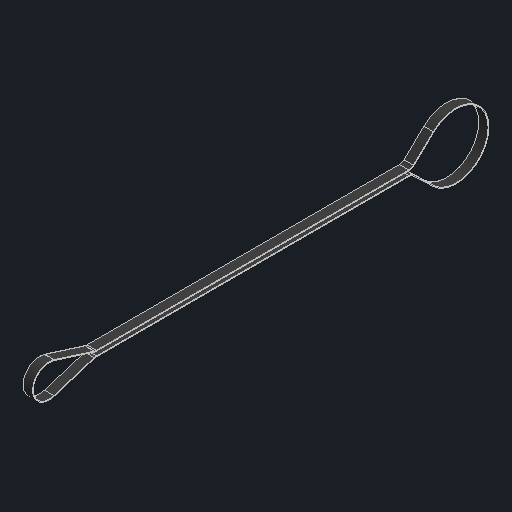
# Autodesk Inventor part: scara-belt3
Saved by Autodesk Inventor 2022 (Build 260153000, 153)
## iProperties
Created: 2021-07-18
Part Number: scara-belt3
Material: ゴム
Document SubType Name: Modeling
Designer: yuta0
Density: 0.93 g/cm^3
Appearance: ゴム - 黒
Mass: 8.55769 g
Surface Area: 248.449 cm^2
Volume: 9.20182 cm^3
Description: 在庫有
購入先: ミスミ
在庫数: 0.0
Author: yuta0
Autodesk Inventor part; units mm, degrees
ref_plane "YZ Plane" through (0, 0, 0) normal (1, 0, 0) x (0, 1, 0)
ref_plane "XZ Plane" through (0, 0, 0) normal (0, 1, 0) x (-1, 0, 0)
ref_plane "XY Plane" through (0, 0, 0) normal (0, 0, 1) x (1, 0, 0)
sketch "スケッチ1" plane through (0, 0, 0) normal (1, 0, 0) x (0, 1, 0)
  arc A0 (16.3891, -5.1817) -> (-16.3891, -5.1817) centre (0, 0) ccw
  arc A1 (-24.8353, -406.9299) -> (24.8353, -406.9299) centre (0, -430.7) ccw
  arc A2 (-2.581, -50) -> (-2.9261, -47.7635) centre (-10, -50) ccw
  line L0 (-2.9261, -47.7635) -> (-16.3891, -5.1817)
  line L1 (16.3891, -5.1817) -> (2.9261, -47.7635)
  line L2 (24.8353, -406.9299) -> (4.6403, -385.8298)
  line L3 (-24.8353, -406.9299) -> (-4.6403, -385.8298)
  arc A3 (2.9261, -47.7635) -> (2.581, -50) centre (10, -50) ccw
  arc A4 (2.581, -380.7) -> (4.6403, -385.8298) centre (10, -380.7) ccw
  arc A5 (-4.6403, -385.8298) -> (-2.581, -380.7) centre (-10, -380.7) ccw
  line L4 (-2.581, -50) -> (-2.581, -380.7)
  line L5 (2.581, -380.7) -> (2.581, -50)
  line L6 (3.3256, -47.8898) -> (16.7886, -5.308)
  arc A6 (16.7886, -5.308) -> (-16.7886, -5.308) centre (0, 0) ccw
  line L7 (-16.7886, -5.308) -> (-3.3256, -47.8898)
  arc A7 (-3, -50) -> (-3.3256, -47.8898) centre (-10, -50) ccw
  line L8 (-3, -50) -> (-3, -380.7)
  arc A8 (-4.943, -385.5401) -> (-3, -380.7) centre (-10, -380.7) ccw
  line L9 (-4.943, -385.5401) -> (-25.138, -406.6402)
  arc A9 (-25.138, -406.6402) -> (25.138, -406.6402) centre (0, -430.7) ccw
  line L10 (25.138, -406.6402) -> (4.943, -385.5401)
  arc A10 (3, -380.7) -> (4.943, -385.5401) centre (10, -380.7) ccw
  line L11 (3, -380.7) -> (3, -50)
  arc A11 (3.3256, -47.8898) -> (3, -50) centre (10, -50) ccw
  arc A12 (2.5629, -47.6486) -> (2.2, -50) centre (10, -50) ccw
  line L12 (2.5629, -47.6486) -> (16.0258, -5.0668)
  arc A13 (16.0258, -5.0668) -> (-16.0258, -5.0668) centre (0, 0) ccw
  line L13 (-16.0258, -5.0668) -> (-2.5629, -47.6486)
  arc A14 (-2.2, -50) -> (-2.5629, -47.6486) centre (-10, -50) ccw
  line L14 (-2.2, -50) -> (-2.2, -380.7)
  arc A15 (-4.365, -386.0933) -> (-2.2, -380.7) centre (-10, -380.7) ccw
  line L15 (-4.365, -386.0933) -> (-24.5601, -407.1934)
  arc A16 (-24.5601, -407.1934) -> (24.5601, -407.1934) centre (0, -430.7) ccw
  line L16 (24.5601, -407.1934) -> (4.365, -386.0933)
  arc A17 (2.2, -380.7) -> (4.365, -386.0933) centre (10, -380.7) ccw
  line L17 (2.2, -380.7) -> (2.2, -50)
  dimension "d0" = 34.3775
  dimension "d1" = 68.7549
  dimension "d2" = 430.7
  dimension "d39" = 0.419
  dimension "d40" = 0.8
  dimension "d41" = 7
  dimension "d42" = 7
  dimension "d43" = 7
  dimension "d44" = 7
  dimension "d45" = 10
  dimension "d46" = 10
  dimension "d47" = 50
  dimension "d48" = 50
  constraints: 36 end point, 36 point on circle, 18 centre point, 12 tangent, 3 vertical alignment, 2 horizontal alignment, 1 coincident, 22 other
  measures "d0" diameter of A0
  measures "d1" diameter of A1
  measures "d2" distance of A0.centre A1.centre
  measures "d39" distance between parallel lines of L11 L5
  measures "d40" distance between parallel lines of L11 L17
  measures "d41" radius of A11
  measures "d42" radius of A7
  measures "d43" radius of A10
  measures "d44" radius of A8
  measures "d45" horizontal distance of point (0, 0) A3.centre
  measures "d46" horizontal distance of point (0, 0) A2.centre
  measures "d47" vertical distance of A1.centre A4.centre
  measures "d48" vertical distance of point (0, 0) A3.centre
extrude "押し出し1" add sketch "スケッチ1" along normal mid plane 10 contours L1 A3 L5 A4 L2 A1 L3 A5 L4 A2 L0 A0 | A11 L11 A10 L10 A9 L9 A8 L8 A7 L7 A6 L6
equation "\"d41\" = d43"
equation "\"d43\" = d44"
equation "\"d44\" = d42"
equation "\"d46\" = d45"
